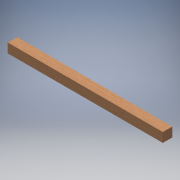
# Autodesk Inventor part: testsideShort
Saved by Autodesk Inventor 2019 (Build 230136000, 136)
## iProperties
Created: 2019-02-01
Part Number: testsideShort
Material: Wood (Cherry)
Document SubType Name: Modeling
Designer: gaincarlo
Density: 0.63 g/cm^3
Appearance: Cherry - Natural Low Gloss
Author: gaincarlo
Autodesk Inventor part; units mm, degrees
ref_plane "YZ Plane" through (0, 0, 0) normal (1, 0, 0) x (0, 1, 0)
ref_plane "XZ Plane" through (0, 0, 0) normal (0, 1, 0) x (-1, 0, 0)
ref_plane "XY Plane" through (0, 0, 0) normal (0, 0, 1) x (1, 0, 0)
sketch "Sketch1" plane through (0, 0, 0) normal (1, 0, 0) x (0, 1, 0)
  line L0 (10, 10) -> (-10, 10)
  line L1 (-10, 10) -> (-10, -10)
  line L2 (-10, -10) -> (10, -10)
  line L3 (10, -10) -> (10, 10)
  line L4 (0, -14) -> (0, 14) projected
  line L5 (-14, 0) -> (14, 0) projected
  point P0 (0, 0)
  point P1 (0, 10)
  point P2 (-10, 0)
  dimension "d0" = 20
  dimension "d1" = 20
  constraints: 8 end point, 2 midpoint, 2 parallel, 2 point on line, 1 horizontal, 1 perpendicular
  measures "d0" distance of L2.end L1.end
  measures "d1" distance of L1.end L0.end
extrude "Extrusion1" add sketch "Sketch1" along normal blind 330
body "Solid1"
